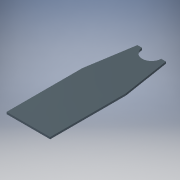
# Autodesk Inventor part: Suporte
Saved by Autodesk Inventor 2016 (Build 200138000, 138)
## iProperties
Created: 2017-04-03
Part Number: Suporte
Material: Lead
Document SubType Name: Modeling
Designer: Marcelo
Mass: 15374 g
Surface Area: 2885.8 cm^2
Volume: 1355.73 cm^3
Density: 11.34 g/cm^3
Appearance: Lead
Author: Marcelo
Autodesk Inventor part; units mm, degrees
ref_plane "YZ Plane" through (0, 0, 0) normal (1, 0, 0) x (0, 1, 0)
ref_plane "XZ Plane" through (0, 0, 0) normal (0, 1, 0) x (-1, 0, 0)
ref_plane "XY Plane" through (0, 0, 0) normal (0, 0, 1) x (1, 0, 0)
sketch "Sketch1" plane through (0, 0, 0) normal (0, 0, 1) x (1, 0, 0)
  line L0 (115, 200) -> (115, -200)
  line L1 (115, -200) -> (-115, -200)
  line L2 (-115, -200) -> (-115, 200)
  arc A0 (-50, 450) -> (50, 450) centre (0, 450) ccw
  line L3 (-115, 200) -> (-75, 450)
  line L4 (75, 450) -> (115, 200)
  line L5 (-75, 450) -> (-50, 450)
  line L6 (50, 450) -> (75, 450)
  point P0 (0, 0)
  dimension "d1" = 400
  dimension "d2" = 115
  dimension "d3" = 200
  dimension "d6" = 100
  dimension "d9" = 150
  dimension "d10" = 25
  dimension "d11" = 25
  dimension "d14" = 450
  dimension "d15" = 230
  dimension "d16" = 170.91
  dimension "d17" = 170.91
  dimension "d18" = 450
  dimension "d19" = 450
  dimension "d20" = 115
  constraints: 14 end point, 2 point on circle, 1 centre point, 1 horizontal, 1 parallel
  measures "d1" distance of L1.end L2.end
  measures "d2" distance from line of point (0, 0) L2
  measures "d3" distance from line of L1 point (0, 0)
  measures "d6" diameter of A0
  measures "d9" distance of L3.end L4.start
  measures "d10" distance of L3.end L5.end
  measures "d11" distance of L6.start L4.start
  measures "d14" distance of point (0, 0) A0.centre
  measures "d15" distance between parallel lines of L2 L0
  measures "d16" angle of L2 L3
  measures "d17" angle of L0 L4
  measures "d18" distance from line of point (0, 0) L5
  measures "d19" distance from line of point (0, 0) L6
  measures "d20" distance from line of L2 A0.centre
extrude "Extrusion1" add sketch "Sketch1" along normal blind 10
equation "\"d2\" = 0.5 * d0"
equation "\"d3\" = 0.5 * d1"
equation "\"d0\" = 230"
body "Solid1"
